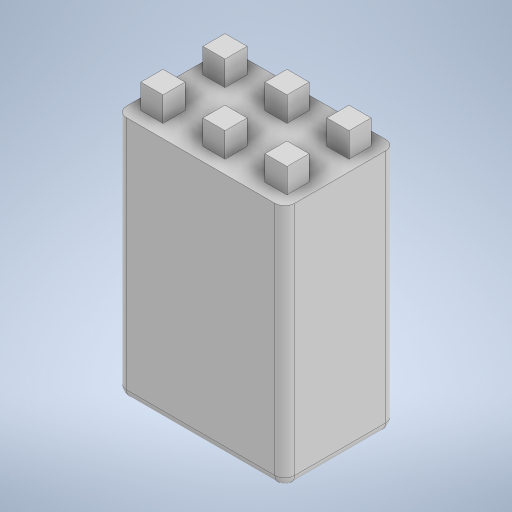
# Autodesk Inventor part: Platform
Saved by Autodesk Inventor 2024 (Build 280153000, 153)
## iProperties
Created: 2024-04-30
Part Number: Platform
Material: Generic
Document SubType Name: Modeling
Designer: cyan924
Density: 1 g/cm^3
Appearance: Default
Author: cyan924
Autodesk Inventor part; units mm, degrees
ref_plane "YZ Plane" through (0, 0, 0) normal (1, 0, 0) x (0, 1, 0)
ref_plane "XZ Plane" through (0, 0, 0) normal (0, 1, 0) x (-1, 0, 0)
ref_plane "XY Plane" through (0, 0, 0) normal (0, 0, 1) x (1, 0, 0)
sketch "Sketch1" plane through (0, 0, 0) normal (0, 1, 0) x (-1, 0, 0)
  line L0 (0, 0) -> (34.2, 0)
  line L1 (34.2, 0) -> (34.2, -22.5)
  line L2 (34.2, -22.5) -> (0, -22.5)
  line L3 (0, -22.5) -> (0, 0)
  line L4 (5, -17.5) -> (29.2, -17.5)
  line L5 (29.2, -17.5) -> (29.2, -5)
  line L6 (29.2, -5) -> (5, -5)
  line L7 (5, -5) -> (5, -17.5)
  dimension "d64" = 24.2
  dimension "d65" = 12.5
  dimension "d66" = 5
  dimension "d67" = 5
  dimension "d68" = 5
  dimension "d69" = 5
  constraints: 16 end point, 4 parallel, 2 horizontal, 2 perpendicular
  measures "d64" distance between parallel lines of L5 L7
  measures "d65" distance of L4.end L5.end
  measures "d66" distance between parallel lines of L1 L5
  measures "d67" distance between parallel lines of L3 L7
  measures "d68" distance between parallel lines of L0 L6
  measures "d69" distance between parallel lines of L2 L4
extrude "Extrusion4" add sketch "Sketch1" along normal blind 16.4
sketch "Sketch6" plane through (0, 16.4, 0) normal (0, 1, 0) x (1, 0, 0)
  line L0 (-34.2, 0) -> (0, 0) projected
  line L1 (0, 22.5) -> (-34.2, 22.5) projected
  line L2 (-34.2, 0) -> (0, 0)
  line L3 (0, 0) -> (0, 22.5)
  line L4 (0, 22.5) -> (-34.2, 22.5)
  line L5 (-34.2, 22.5) -> (-34.2, 0)
  constraints: 8 end point, 2 parallel, 1 horizontal, 1 perpendicular
extrude "Extrusion6" add sketch "Sketch6" along normal blind 33.5
sketch "Sketch8" plane through (-34.2, 0, -22.5) normal (-1, 0, 0) x (0, 0, 1)
  line L0 (17.5, 0) -> (17.5, 16.4) projected
  line L1 (5, 16.4) -> (17.5, 16.4) projected
  line L2 (17.5, 6.4) -> (5, 6.4)
  line L3 (5, 6.4) -> (5, 16.4)
  line L4 (5, 16.4) -> (17.5, 16.4)
  line L5 (17.5, 16.4) -> (17.5, 6.4)
  point P0 (22.5, 0)
  dimension "d176" = 10
  constraints: 8 end point, 2 parallel, 1 horizontal, 1 perpendicular, 1 point on line
  measures "d176" distance between parallel lines of L1 L2
extrude "Extrusion8" cut sketch "Sketch8" against normal blind 7.5
fillet "Fillet2" radius 2 11 edges at (-17.1, 0, -22.5) (-34.2, 0, -11.25) (0, 0, -11.25) (-17.1, 0, 0) (0, 24.95, -22.5) (0, 24.95, 0) (-34.2, 24.95, -22.5) (-34.2, 24.95, 0) (-34.2, 11.4, -5) (-34.2, 6.4, -11.25) (-34.2, 11.4, -17.5)
sketch "Sketch9" plane through (0, 49.9, 0) normal (0, 1, 0) x (1, 0, 0)
  line L0 (-2, 22.5) -> (-32.2, 22.5) construction
  line L1 (-17.1, 22.5) -> (-17.1, 0) construction
  line L2 (-34.2, 2) -> (-34.2, 20.5) construction
  line L3 (-34.2, 11.25) -> (0, 11.25) construction
  line L4 (0, 20.5) -> (0, 2) construction
  line L5 (-17.1, 11.25) -> (-17.1, 15.3) construction
  line L6 (-17.1, 15.3) -> (-14.85, 15.3) construction
  line L7 (-17.1, 11.25) -> (-17.1, 7.2) construction
  line L8 (-17.1, 7.2) -> (-14.85, 7.2) construction
  line L9 (-14.85, 7.2) -> (-19.35, 7.2)
  line L10 (-19.35, 7.2) -> (-19.35, 2.7)
  line L11 (-19.35, 2.7) -> (-14.85, 2.7)
  line L12 (-14.85, 2.7) -> (-14.85, 7.2)
  line L13 (-14.85, 15.3) -> (-19.35, 15.3)
  line L14 (-19.35, 15.3) -> (-19.35, 19.8)
  line L15 (-19.35, 19.8) -> (-14.85, 19.8)
  line L16 (-14.85, 19.8) -> (-14.85, 15.3)
  line L17 (-19.35, 15.3) -> (-27.45, 15.3) construction
  line L18 (-19.35, 2.7) -> (-27.45, 2.7) construction
  line L19 (-14.85, 2.7) -> (-6.75, 2.7) construction
  line L20 (-14.85, 15.3) -> (-6.75, 15.3) construction
  line L21 (-27.45, 15.3) -> (-31.95, 15.3)
  line L22 (-31.95, 15.3) -> (-31.95, 19.8)
  line L23 (-31.95, 19.8) -> (-27.45, 19.8)
  line L24 (-27.45, 19.8) -> (-27.45, 15.3)
  line L25 (-27.45, 2.7) -> (-31.95, 2.7)
  line L26 (-31.95, 2.7) -> (-31.95, 7.2)
  line L27 (-31.95, 7.2) -> (-27.45, 7.2)
  line L28 (-27.45, 7.2) -> (-27.45, 2.7)
  line L29 (-6.75, 2.7) -> (-2.25, 2.7)
  line L30 (-2.25, 2.7) -> (-2.25, 7.2)
  line L31 (-2.25, 7.2) -> (-6.75, 7.2)
  line L32 (-6.75, 7.2) -> (-6.75, 2.7)
  line L33 (-6.75, 15.3) -> (-2.25, 15.3)
  line L34 (-2.25, 15.3) -> (-2.25, 19.8)
  line L35 (-2.25, 19.8) -> (-6.75, 19.8)
  line L36 (-6.75, 19.8) -> (-6.75, 15.3)
  point P0 (0, 0)
  dimension "d180" = 4.05
  dimension "d181" = 2.25
  dimension "d182" = 4.05
  dimension "d183" = 2.25
  dimension "d184" = 4.5
  dimension "d185" = 4.5
  dimension "d186" = 4.5
  dimension "d187" = 4.5
  dimension "d188" = 8.1
  dimension "d189" = 8.1
  dimension "d190" = 8.1
  dimension "d191" = 8.1
  dimension "d192" = 4.5
  dimension "d193" = 4.5
  dimension "d194" = 4.5
  dimension "d195" = 4.5
  dimension "d196" = 4.5
  dimension "d197" = 4.5
  dimension "d198" = 4.5
  dimension "d199" = 4.5
  constraints: 68 end point, 12 parallel, 9 perpendicular, 7 horizontal, 4 midpoint, 2 point on line, 1 vertical
  measures "d180" distance of L5.start L5.end
  measures "d181" distance of L5.end L6.end
  measures "d182" distance of L5.start L7.end
  measures "d183" distance of L7.end L8.end
  measures "d184" distance of L11.end L10.end
  measures "d185" distance of L10.end L9.end
  measures "d186" distance of L14.end L15.end
  measures "d187" distance of L13.end L14.end
  measures "d188" distance of L13.end L17.end
  measures "d189" distance of L10.end L18.end
  measures "d190" distance of L11.end L19.end
  measures "d191" distance of L6.end L20.end
  measures "d192" distance of L22.end L23.end
  measures "d193" distance of L21.end L22.end
  measures "d194" distance of L26.end L27.end
  measures "d195" distance of L25.end L26.end
  measures "d196" distance of L31.end L30.end
  measures "d197" distance of L30.end L29.end
  measures "d198" distance of L35.end L34.end
  measures "d199" distance of L34.end L33.end
extrude "Extrusion9" add sketch "Sketch9" along normal blind 5
equation "\"box\" = 4.5"
equation "\"walllength\" = 1"
equation "\"gap\" = 8.1"
equation "\"d34\" = 4.6"
equation "\"d35\" = 8"
equation "\"offset\" = 5"
equation "\"d44\" = 4.6"
equation "\"d89\" = 4.6"
equation "\"d126\" = 4.6"
equation "\"d134\" = 4.6"
equation "\"d135\" = 8"
equation "\"d140\" = 4.6"
equation "\"d144\" = 4.6"
equation "\"d162\" = 4.6"
equation "\"d163\" = 4.6"
equation "\"d164\" = 8"
equation "\"d165\" = 4.6"
equation "\"d166\" = 4.6"
equation "\"d167\" = 4.6"
body "Solid2"
